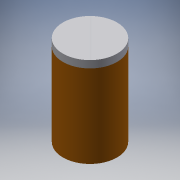
# Autodesk Inventor part: Tun-Placeholder
Saved by Autodesk Inventor 2017 (Build 210142000, 142)
## iProperties
Created: 2017-08-30
Part Number: Tun-Placeholder
Material: Generic
Document SubType Name: Modeling
Designer: Trent
Density: 1 g/cm^3
Appearance: Default
Author: Trent
Autodesk Inventor part; units mm, degrees
ref_plane "YZ Plane" through (0, 0, 0) normal (1, 0, 0) x (0, 1, 0)
ref_plane "XZ Plane" through (0, 0, 0) normal (0, 1, 0) x (-1, 0, 0)
ref_plane "XY Plane" through (0, 0, 0) normal (0, 0, 1) x (1, 0, 0)
sketch "Sketch1" plane through (0, 0, 0) normal (0, 1, 0) x (-1, 0, 0)
  circle A0 centre (0, 0) radius 190.5
  dimension "d0" = 381
  constraints: 1 centre point, 1 coincident
  measures "d0" diameter of A0
extrude "Extrusion1" add sketch "Sketch1" along normal blind 25.4
sketch "Sketch2" plane through (0, 25.4, 0) normal (0, 1, 0) x (1, 0, 0)
  circle A0 centre (0, 0) radius 177.8
  circle A1 centre (0, 0) radius 190.5 projected
  dimension "d3" = 355.6
  constraints: 1 centre point, 1 coincident
  measures "d3" diameter of A0
extrude "Extrusion2" add sketch "Sketch2" along normal blind 558.8
sketch "Sketch3" plane through (0, 584.2, 0) normal (0, 1, 0) x (1, 0, 0)
  circle A0 centre (0, 0) radius 190.8969
  dimension "d6" = 381.7937
  constraints: 1 centre point, 1 coincident
  measures "d6" diameter of A0
extrude "Extrusion3" add sketch "Sketch3" along normal blind 50.8
ref_plane "Work Plane2" through (190.5, 0, 0) normal (1, 0, 0) x (0, 1, 0)
ref_plane "Work Plane1" through (228.6, -12.7, -4375.1201) normal (1, 0, 0) x (0, 1, 0)
ref_plane "Work Plane4" through (0, 0, 190.5) normal (0, 0, 1) x (1, 0, 0)
ref_plane "Work Plane3" through (-228.6, -12.7, 203.2) normal (0, 0, 1) x (1, 0, 0)
body "Solid1"
